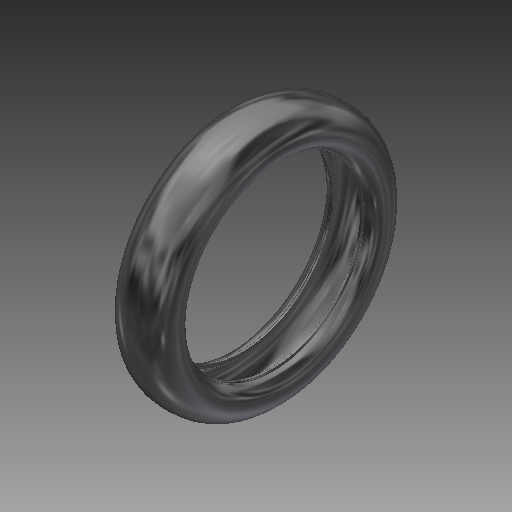
# Autodesk Inventor part: Opona_koła_przedniego
Saved by Autodesk Inventor 2017 (Build 210142000, 142)
## iProperties
Created: 2015-12-01
Part Number: Opona_koła_przedniego
Material: Kauczuk, silikon
Document SubType Name: Modeling
Designer: graaapsik
Density: 1.25 g/cm^3
Appearance: Kauczuk - czarny - wersja 1.1
Mass: 62.0028 g
Surface Area: 506.663 cm^2
Volume: 49.6023 cm^3
Author: graaapsik
Autodesk Inventor part; units mm, degrees
ref_plane "YZ Plane" through (0, 0, 0) normal (1, 0, 0) x (0, 1, 0)
ref_plane "XZ Plane" through (0, 0, 0) normal (0, 1, 0) x (-1, 0, 0)
ref_plane "Płaszczyzna konstrukcyjna3" through (101.853418, 8.018249, 49.010933) normal (0, 0.265026, -0.9642413) x (1, 0, 0)
sketch "Szkic4" plane through (101.853418, 8.018249, 49.010933) normal (0, 0.265026, -0.9642413) x (1, 0, 0)
  line L0 (-12.35, 51) -> (-9.754164, 51) construction
  line L1 (-9.179631, 50.732091) -> (-8.883022, 50.378606) construction
  line L2 (-8.5, 50.2) -> (-6.875, 50.2) construction
  arc A0 (-8.883022, 50.378606) -> (-8.5, 50.2) centre (-8.5, 50.7) ccw construction
  arc A1 (-9.179631, 50.732091) -> (-9.754164, 51) centre (-9.754164, 50.25) ccw construction
  line L3 (-9.171971, 50.738519) -> (-8.811405, 50.308814)
  arc A2 (-9.171971, 50.738519) -> (-9.734965, 51.009757) centre (-9.754164, 50.25) ccw
  arc A3 (-10.329351, 51.11595) -> (-9.734965, 51.009757) centre (-9.68444, 53.009119) ccw
  arc A4 (-10.329351, 51.11595) -> (-11.035486, 51.35) centre (-24.839852, 8.519643) ccw
  arc A5 (-15.874455, 58.45) -> (-11.035486, 51.35) centre (-8.888141, 58.0125) ccw
  arc A6 (-8.693747, 68.7) -> (-15.874455, 58.45) centre (-3.897916, 57.7) ccw
  arc A7 (-1.5, 70.2) -> (-8.693747, 68.7) centre (-1.5, 52.2) ccw
  line L4 (-4.165584, 57.749949) -> (4.277424, 57.749949) construction
  line L5 (-1.5, 70.2) -> (0, 70.2)
  arc A8 (-8.811405, 50.308814) -> (-8.5, 50.2) centre (-8.5, 50.7) ccw
  line L6 (-8.5, 50.2) -> (-7.821047, 50.2)
  arc A9 (-7.821047, 50.2) -> (-7.671047, 50.35) centre (-7.821047, 50.35) ccw
  line L7 (-7.671047, 50.35) -> (-7.671047, 52.016429)
  arc A10 (-7.671047, 52.016429) -> (-8.707229, 53.015774) centre (-8.671047, 52.016429) ccw
  line L8 (-8.47801, 50.43531) -> (-8.5, 50.43531)
  arc A11 (-9.684439, 53.009099) -> (-9.684441, 53.009099) centre (-9.68444, 53.009119) ccw
  arc A12 (-13.878365, 58.325) -> (-8.707229, 53.015774) centre (-8.888141, 58.0125) ccw
  arc A13 (-7.894442, 66.866667) -> (-13.878365, 58.325) centre (-3.897916, 57.7) ccw
  arc A14 (-1.5, 68.2) -> (-7.894442, 66.866667) centre (-1.5, 52.2) ccw
  line L9 (-1.5, 68.2) -> (0, 68.2)
  line L10 (-12.5, -50.85) -> (-12.5, 50.85) construction
  line L11 (12.5, -50.85) -> (12.5, 50.85) construction
  line L12 (37.5, 47.263297) -> (37.5, 53.920969) construction
  line L13 (-37.5, 51.183214) -> (-37.5, 44.81995) construction
  line L14 (0, 70.947992) -> (0, 46.303819) construction
  line L15 (12.35, 51) -> (9.754164, 51) construction
  line L16 (9.179631, 50.732091) -> (8.883022, 50.378606) construction
  line L17 (8.5, 50.2) -> (6.875, 50.2) construction
  arc A15 (8.5, 50.2) -> (8.883022, 50.378606) centre (8.5, 50.7) ccw construction
  arc A16 (9.754164, 51) -> (9.179631, 50.732091) centre (9.754164, 50.25) ccw construction
  line L18 (9.171971, 50.738519) -> (8.811405, 50.308814)
  arc A17 (9.734965, 51.009757) -> (9.171971, 50.738519) centre (9.754164, 50.25) ccw
  arc A18 (9.734965, 51.009757) -> (10.329351, 51.11595) centre (9.68444, 53.009119) ccw
  arc A19 (11.035486, 51.35) -> (10.329351, 51.11595) centre (24.839852, 8.519643) ccw
  arc A20 (11.035486, 51.35) -> (15.874455, 58.45) centre (8.888141, 58.0125) ccw
  arc A21 (15.874455, 58.45) -> (8.693747, 68.7) centre (3.897916, 57.7) ccw
  arc A22 (8.693747, 68.7) -> (1.5, 70.2) centre (1.5, 52.2) ccw
  line L19 (1.5, 70.2) -> (0, 70.2)
  arc A23 (8.5, 50.2) -> (8.811405, 50.308814) centre (8.5, 50.7) ccw
  line L20 (8.5, 50.2) -> (7.821047, 50.2)
  arc A24 (7.671047, 50.35) -> (7.821047, 50.2) centre (7.821047, 50.35) ccw
  line L21 (7.671047, 50.35) -> (7.671047, 52.016429)
  arc A25 (8.707229, 53.015774) -> (7.671047, 52.016429) centre (8.671047, 52.016429) ccw
  line L22 (8.47801, 50.43531) -> (8.5, 50.43531)
  arc A26 (9.684441, 53.009099) -> (9.684439, 53.009099) centre (9.68444, 53.009119) ccw
  arc A27 (8.707229, 53.015774) -> (13.878365, 58.325) centre (8.888141, 58.0125) ccw
  arc A28 (13.878365, 58.325) -> (7.894442, 66.866667) centre (3.897916, 57.7) ccw
  arc A29 (7.894442, 66.866667) -> (1.5, 68.2) centre (1.5, 52.2) ccw
  line L23 (1.5, 68.2) -> (0, 68.2)
  line L24 (-31.5, 0) -> (31.5, 0) construction
  point P0 (4.165584, 57.749949)
  dimension "d0" = 0.01
  dimension "d1" = 20
  dimension "d2" = 2
  dimension "d3" = 18
  dimension "d4" = 12
  dimension "d5" = 7
  dimension "d6" = 2
  dimension "d7" = 0.76
  dimension "d8" = 0.5
  dimension "d9" = 0.15
  dimension "d11" = 1.5
  dimension "d12" = 11.75
  dimension "d13" = 1
  dimension "d15" = 2.81577
  dimension "d19" = 1.5
  dimension "d20" = 1.5
  dimension "d21" = 45
  dimension "d22" = 0.35
  constraints: 60 point on circle, 46 end point, 40 symmetric about line, 30 centre point, 11 tangent, 9 parallel, 4 horizontal, 2 point on line, 1 perpendicular, 37 other
  measures "d0" distance between parallel lines of L3 L1
  measures "d1" distance between parallel lines of L5 L2
  measures "d2" radial gap between concentric circles of A12 A5
  measures "d3" radius of A7
  measures "d4" radius of A6
  measures "d5" radius of A5
  measures "d6" radius of A3
  measures "d7" radius of A2
  measures "d8" radius of A8
  measures "d9" radius of A9
  measures "d11" distance from line of A6.start L5
  measures "d12" distance from line of A5.start L5
  measures "d13" radius of A10
  measures "d15" distance from line of A10.end L2
  measures "d19" distance of L5.start L5.end
  measures "d20" distance of L9.start L9.end
  measures "d21" radius of A4
  measures "d22" distance from line of L0 A4.end
sketch "Szkic4 outline for Obrót1" plane through (101.853418, 8.018249, 49.010933) normal (0, 0.265026, -0.9642413) x (1, 0, 0)
  arc A0 (-9.734965, 51.009757) -> (-9.171971, 50.738519) centre (-9.754164, 50.25) cw
  arc A1 (-10.329351, 51.11595) -> (-9.734965, 51.009757) centre (-9.68444, 53.009119) ccw
  arc A2 (-11.035486, 51.35) -> (-10.329351, 51.11595) centre (-24.839852, 8.519643) cw
  arc A3 (-15.874455, 58.45) -> (-11.035486, 51.35) centre (-8.888141, 58.0125) ccw
  arc A4 (-8.693747, 68.7) -> (-15.874455, 58.45) centre (-3.897916, 57.7) ccw
  arc A5 (-1.5, 70.2) -> (-8.693747, 68.7) centre (-1.5, 52.2) ccw
  line L0 (0, 70.2) -> (-1.5, 70.2)
  line L1 (1.5, 70.2) -> (0, 70.2)
  arc A6 (8.693747, 68.7) -> (1.5, 70.2) centre (1.5, 52.2) ccw
  arc A7 (15.874455, 58.45) -> (8.693747, 68.7) centre (3.897916, 57.7) ccw
  arc A8 (11.035486, 51.35) -> (15.874455, 58.45) centre (8.888141, 58.0125) ccw
  arc A9 (10.329351, 51.11595) -> (11.035486, 51.35) centre (24.839852, 8.519643) cw
  arc A10 (9.734965, 51.009757) -> (10.329351, 51.11595) centre (9.68444, 53.009119) ccw
  arc A11 (9.171971, 50.738519) -> (9.734965, 51.009757) centre (9.754164, 50.25) cw
  line L2 (8.811405, 50.308814) -> (9.171971, 50.738519)
  arc A12 (8.5, 50.2) -> (8.811405, 50.308814) centre (8.5, 50.7) ccw
  line L3 (7.821047, 50.2) -> (8.5, 50.2)
  arc A13 (7.671047, 50.35) -> (7.821047, 50.2) centre (7.821047, 50.35) ccw
  line L4 (7.671047, 52.016429) -> (7.671047, 50.35)
  arc A14 (8.707229, 53.015774) -> (7.671047, 52.016429) centre (8.671047, 52.016429) ccw
  arc A15 (13.878365, 58.325) -> (8.707229, 53.015774) centre (8.888141, 58.0125) cw
  arc A16 (7.894442, 66.866667) -> (13.878365, 58.325) centre (3.897916, 57.7) cw
  arc A17 (1.5, 68.2) -> (7.894442, 66.866667) centre (1.5, 52.2) cw
  line L5 (0, 68.2) -> (1.5, 68.2)
  line L6 (-1.5, 68.2) -> (0, 68.2)
  arc A18 (-7.894442, 66.866667) -> (-1.5, 68.2) centre (-1.5, 52.2) cw
  arc A19 (-13.878365, 58.325) -> (-7.894442, 66.866667) centre (-3.897916, 57.7) cw
  arc A20 (-8.707229, 53.015774) -> (-13.878365, 58.325) centre (-8.888141, 58.0125) cw
  arc A21 (-7.671047, 52.016429) -> (-8.707229, 53.015774) centre (-8.671047, 52.016429) ccw
  line L7 (-7.671047, 50.35) -> (-7.671047, 52.016429)
  arc A22 (-7.821047, 50.2) -> (-7.671047, 50.35) centre (-7.821047, 50.35) ccw
  line L8 (-8.5, 50.2) -> (-7.821047, 50.2)
  arc A23 (-8.811405, 50.308814) -> (-8.5, 50.2) centre (-8.5, 50.7) ccw
  line L9 (-9.171971, 50.738519) -> (-8.811405, 50.308814)
revolve "Obrót1" add sketch "Szkic4 outline for Obrót1" angle 360 about axis through (70.353418, 8.018249, 49.010933) along (1, 0, 0)
